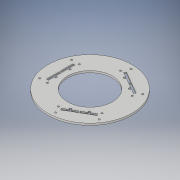
# Autodesk Inventor part: Stewart-Platform-Base-Außenanordnung
Saved by Autodesk Inventor 2018.2 (Build 222227000, 227)
## iProperties
Created: 2018-02-17
Part Number: Stewart-Platform-Base-Außenanordnung
Material: Generisch
Document SubType Name: Modeling
Designer: JochenAlt
Density: 1 g/cm^3
Appearance: Vorgabe
Author: JochenAlt
Autodesk Inventor part; units mm, degrees
ref_plane "YZ Plane" through (0, 0, 0) normal (1, 0, 0) x (0, 1, 0)
ref_plane "XZ Plane" through (0, 0, 0) normal (0, 1, 0) x (-1, 0, 0)
ref_plane "XY Plane" through (0, 0, 0) normal (0, 0, 1) x (1, 0, 0)
sketch "Skizze1" plane through (0, 0, 0) normal (0, 0, 1) x (1, 0, 0)
  line L0 (0, 94.6756) -> (0, -94.6756) construction
  line L1 (-94.6756, 0) -> (94.6756, 0) construction
  line L2 (-55.2629, 29.05) -> (-42.8629, 29.05) construction
  line L3 (-39.4629, 25.65) -> (-39.4629, -25.65) construction
  line L4 (-42.8629, -29.05) -> (-55.2629, -29.05) construction
  line L5 (-58.6629, -25.65) -> (-58.6629, 25.65) construction
  arc A0 (-55.2629, 29.05) -> (-58.6629, 25.65) centre (-55.2629, 25.65) ccw construction
  arc A1 (-39.4629, 25.65) -> (-42.8629, 29.05) centre (-42.8629, 25.65) ccw construction
  arc A2 (-42.8629, -29.05) -> (-39.4629, -25.65) centre (-42.8629, -25.65) ccw construction
  arc A3 (-58.6629, -25.65) -> (-55.2629, -29.05) centre (-55.2629, -25.65) ccw construction
  circle A4 centre (-55.2629, 25.65) radius 1.4
  circle A5 centre (-42.8629, 25.65) radius 1.4
  circle A6 centre (-55.2629, -25.65) radius 1.4
  circle A7 centre (-42.8629, -25.65) radius 1.4
  line L6 (-45.3629, 21.4) -> (-45.3629, -21.4)
  line L7 (-48.6629, 21.4) -> (-48.6629, -21.4)
  line L8 (-48.6629, 21.4) -> (-45.3629, 21.4)
  line L9 (-48.6629, -21.4) -> (-45.3629, -21.4)
  line L10 (-48.6629, 0.8) -> (-45.3629, 0.8)
  line L11 (-48.6629, -0.8) -> (-45.3629, -0.8)
  line L12 (-45.3629, 12.5) -> (-42.4469, 12.5)
  line L13 (-42.4469, 12.5) -> (-42.4469, 9.7)
  line L14 (-42.4469, 9.7) -> (-45.3629, 9.7)
  line L15 (-45.3629, -9.7) -> (-42.4469, -9.7)
  line L16 (-42.4469, -9.7) -> (-42.4469, -12.5)
  line L17 (-42.4469, -12.5) -> (-45.3629, -12.5)
  line L18 (-42.8629, 29.35) -> (-55.2629, 29.35)
  arc A8 (-55.2629, 29.35) -> (-58.9629, 25.65) centre (-55.2629, 25.65) ccw
  line L19 (-58.9629, 25.65) -> (-58.9629, -25.65)
  arc A9 (-58.9629, -25.65) -> (-55.2629, -29.35) centre (-55.2629, -25.65) ccw
  line L20 (-55.2629, -29.35) -> (-42.8629, -29.35)
  arc A10 (-42.8629, -29.35) -> (-39.1629, -25.65) centre (-42.8629, -25.65) ccw
  line L21 (-39.1629, -25.65) -> (-39.1629, 25.65)
  arc A11 (-39.1629, 25.65) -> (-42.8629, 29.35) centre (-42.8629, 25.65) ccw
  line L22 (-61.0807, -28.9731) -> (-58.4757, -27.4852) construction
  line L23 (42.8644, -31.4433) -> (41.2144, -28.5854)
  circle A12 centre (43.645, -24.2953) radius 1.4
  arc A13 (46.5895, -22.5953) -> (41.945, -21.3508) centre (43.645, -24.2953) ccw construction
  arc A14 (46.8493, -22.4453) -> (41.795, -21.091) centre (43.645, -24.2953) ccw
  circle A15 centre (49.845, -35.034) radius 1.4
  line L24 (55.6318, -38.4109) -> (53.0407, -36.8988) construction
  arc A16 (51.545, -37.9785) -> (52.7895, -33.334) centre (49.845, -35.034) ccw construction
  arc A17 (51.695, -38.2383) -> (53.0493, -33.184) centre (49.845, -35.034) ccw
  line L25 (53.0493, -33.184) -> (46.8493, -22.4453)
  line L26 (46.5895, -22.5953) -> (52.7895, -33.334) construction
  line L27 (2.4734, -62.384) -> (-3.7266, -51.6453) construction
  arc A18 (2.4734, -62.384) -> (7.1179, -63.6285) centre (5.4179, -60.684) ccw construction
  circle A19 centre (5.4179, -60.684) radius 1.4
  circle A20 centre (-0.7821, -49.9453) radius 1.4
  arc A21 (2.2136, -62.534) -> (7.2679, -63.8883) centre (5.4179, -60.684) ccw
  line L28 (-3.9864, -51.7953) -> (2.2136, -62.534)
  arc A22 (-2.4821, -47.0008) -> (-3.7266, -51.6453) centre (-0.7821, -49.9453) ccw construction
  arc A23 (-2.6321, -46.741) -> (-3.9864, -51.7953) centre (-0.7821, -49.9453) ccw
  line L29 (32.0487, -30.5101) -> (33.5067, -33.0354)
  line L30 (29.6239, -31.9101) -> (32.0487, -30.5101)
  line L31 (31.0819, -34.4354) -> (29.6239, -31.9101)
  line L32 (5.7985, -52.8433) -> (4.1485, -49.9854)
  line L33 (11.8561, -45.5354) -> (10.3981, -43.0101)
  line L34 (10.3981, -43.0101) -> (12.823, -41.6101)
  line L35 (12.823, -41.6101) -> (14.281, -44.1354)
  line L36 (23.6386, -42.5433) -> (21.9886, -39.6854)
  line L37 (25.0242, -41.7433) -> (23.3742, -38.8854)
  line L38 (4.1485, -49.9854) -> (41.2144, -28.5854)
  line L39 (41.795, -21.091) -> (-2.6321, -46.741)
  line L40 (-2.4821, -47.0008) -> (41.945, -21.3508) construction
  line L41 (51.545, -37.9785) -> (7.1179, -63.6285) construction
  line L42 (7.2679, -63.8883) -> (51.695, -38.2383)
  line L43 (5.7985, -52.8433) -> (42.8644, -31.4433)
  line L44 (5.7985, 52.8433) -> (4.1485, 49.9854)
  circle A24 centre (-0.7821, 49.9453) radius 1.4
  arc A25 (-3.7266, 51.6453) -> (-2.4821, 47.0008) centre (-0.7821, 49.9453) ccw construction
  arc A26 (-3.9864, 51.7953) -> (-2.6321, 46.741) centre (-0.7821, 49.9453) ccw
  circle A27 centre (5.4179, 60.684) radius 1.4
  line L45 (5.4489, 67.384) -> (5.435, 64.384) construction
  arc A28 (7.1179, 63.6285) -> (2.4734, 62.384) centre (5.4179, 60.684) ccw construction
  arc A29 (7.2679, 63.8883) -> (2.2136, 62.534) centre (5.4179, 60.684) ccw
  line L46 (2.2136, 62.534) -> (-3.9864, 51.7953)
  line L47 (-3.7266, 51.6453) -> (2.4734, 62.384) construction
  line L48 (52.7895, 33.334) -> (46.5895, 22.5953) construction
  arc A30 (52.7895, 33.334) -> (51.545, 37.9785) centre (49.845, 35.034) ccw construction
  circle A31 centre (49.845, 35.034) radius 1.4
  circle A32 centre (43.645, 24.2953) radius 1.4
  arc A33 (53.0493, 33.184) -> (51.695, 38.2383) centre (49.845, 35.034) ccw
  line L49 (46.8493, 22.4453) -> (53.0493, 33.184)
  arc A34 (41.945, 21.3508) -> (46.5895, 22.5953) centre (43.645, 24.2953) ccw construction
  arc A35 (41.795, 21.091) -> (46.8493, 22.4453) centre (43.645, 24.2953) ccw
  line L50 (10.3981, 43.0101) -> (11.8561, 45.5354)
  line L51 (12.823, 41.6101) -> (10.3981, 43.0101)
  line L52 (14.281, 44.1354) -> (12.823, 41.6101)
  line L53 (42.8644, 31.4433) -> (41.2144, 28.5854)
  line L54 (33.5067, 33.0354) -> (32.0487, 30.5101)
  line L55 (32.0487, 30.5101) -> (29.6239, 31.9101)
  line L56 (29.6239, 31.9101) -> (31.0819, 34.4354)
  line L57 (25.0242, 41.7433) -> (23.3742, 38.8854)
  line L58 (23.6386, 42.5433) -> (21.9886, 39.6854)
  line L59 (41.2144, 28.5854) -> (4.1485, 49.9854)
  line L60 (-2.6321, 46.741) -> (41.795, 21.091)
  line L61 (41.945, 21.3508) -> (-2.4821, 47.0008) construction
  line L62 (7.1179, 63.6285) -> (51.545, 37.9785) construction
  line L63 (51.695, 38.2383) -> (7.2679, 63.8883)
  line L64 (42.8644, 31.4433) -> (5.7985, 52.8433)
  line L65 (-36.1629, 0) -> (-39.1629, 0) construction
  circle A36 centre (0, 0) radius 36.1629
  circle A37 centre (0, 0) radius 67.6254
  line L66 (-61.3401, 28.4707) -> (-58.619, 27.2077) construction
  line L67 (-42.4469, -11.1) -> (-6.4086, -11.1) construction
  line L68 (11.6105, -42.3101) -> (-6.4086, -11.1) construction
  line L69 (-38.1629, -11.1) -> (-38.1629, -66.1) construction
  line L70 (9.4685, -38.6) -> (-38.1629, -66.1) construction
  dimension "d43" = 135.2508
  dimension "d1" = 58.1
  dimension "d2" = 19.2
  dimension "d3" = 3.4
  dimension "d5" = 2.8
  dimension "d6" = 5.9
  dimension "d7" = 3.3
  dimension "d8" = 20.6
  dimension "d9" = 1.6
  dimension "d10" = 2.984
  dimension "d11" = 2.8
  dimension "d12" = 19.4
  dimension "d21" = 0.3
  dimension "d22" = 3
  dimension "d32" = 360
  dimension "d34" = 3
  dimension "d35" = 3
  dimension "d40" = 1
  dimension "d41" = 1
  dimension "d42" = 55
  constraints: 138 end point, 52 point on circle, 36 centre point, 27 point on line, 14 coincident, 9 perpendicular, 8 tangent, 7 horizontal, 6 equal radius, 4 midpoint, 4 parallel, 3 vertical, 2 line through centre, 1 collinear, 1 horizontal alignment, 244 other
  measures "d1" distance between parallel lines of L4 L2
  measures "d2" distance between parallel lines of L3 L5
  measures "d3" radius of A0
  measures "d5" diameter of A4
  measures "d6" distance between parallel lines of L3 L6
  measures "d7" distance between parallel lines of L6 L7
  measures "d8" distance between parallel lines of L10 L8
  measures "d9" distance between parallel lines of L11 L10
  measures "d10" distance between parallel lines of L3 L13
  measures "d11" distance between parallel lines of L14 L12
  measures "d12" distance between parallel lines of L15 L14
  measures "d21" distance between parallel lines of L19 L5
  measures "d22" distance of L22.end L22.start
  measures "d34" distance of L65.start L65.end
  measures "d35" distance of L66.start L66.end
  measures "d40" distance between parallel lines of L21 L69
  measures "d41" distance between parallel lines of L70 L39
  measures "d42" distance from line of L67 L69.end
extrude "Extrusion5" add sketch "Skizze1" along normal blind 3 contours L10 L6 L11 L7 | A11 L21 A10 L20 A9 L19 A8 L18 | L43 L36 L38 L37 | L25 A17 L42 A21 L28 A23 L39 A14 | L64 L57 L59 L58 | L46 A29 L63 A33 L49 A35 L60 A26 | A37
extrude "Extrusion4" cut sketch "Skizze1" along normal blind 1 contours L10 L6 L11 L7 | A11 L21 A10 L20 A9 L19 A8 L18 | L43 L36 L38 L37 | L25 A17 L42 A21 L28 A23 L39 A14 | L64 L57 L59 L58 | L46 A29 L63 A33 L49 A35 L60 A26
equation "\"d22\" = d20"
equation "\"d35\" = d34"
equation "\"d41\" = d40"
equation "\"d20\" = 3"
